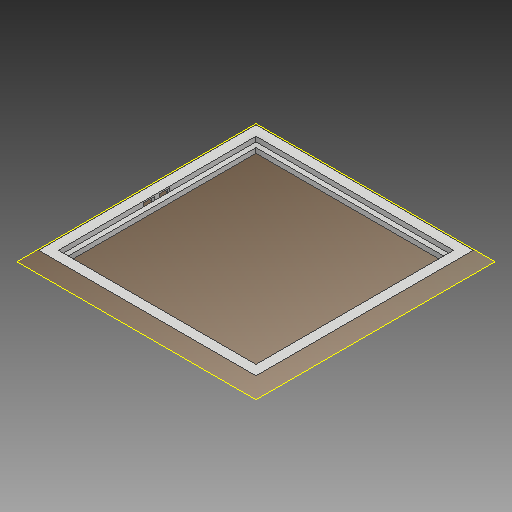
# Autodesk Inventor part: PV_Ramen_CPY
Saved by Autodesk Inventor 2018.2 (Build 222227000, 227)
## iProperties
Created: 2019-09-06
Part Number: PV_Ramen_CPY
Material: Generisch
Document SubType Name: Modeling
Designer: Lolob
Density: 1 g/cm^3
Appearance: Vorgabe
Author: DerLobre
Autodesk Inventor part; units mm, degrees
ref_plane "YZ Plane" through (0, 0, 0) normal (1, 0, 0) x (0, 1, 0)
ref_plane "XZ Plane" through (0, 0, 0) normal (0, 1, 0) x (-1, 0, 0)
ref_plane "XY Plane" through (0, 0, 0) normal (0, 0, 1) x (1, 0, 0)
sketch "Skizze1" plane through (0, 0, 0) normal (0, 0, 1) x (1, 0, 0)
  line L0 (-220, -220) -> (220, -220) projected
  line L1 (220, 220) -> (220, -220) projected
  line L2 (-220, 220) -> (-220, -220) projected
  line L3 (-220, 220) -> (220, 220) projected
  line L4 (200, 200) -> (-200, 200) projected
  line L5 (-200, 200) -> (-200, -200) projected
  line L6 (-200, -200) -> (200, -200) projected
  line L7 (200, -200) -> (200, 200) projected
  line L8 (220, -220) -> (-220, -220)
  line L9 (-220, -220) -> (-220, 220)
  line L10 (-220, 220) -> (220, 220)
  line L11 (220, 220) -> (220, -220)
  line L12 (200, -200) -> (-200, -200)
  line L13 (-200, -200) -> (-200, 200)
  line L14 (-200, 200) -> (200, 200)
  line L15 (200, 200) -> (200, -200)
  point P0 (0, 0)
  constraints: 16 end point, 4 parallel, 2 horizontal, 2 perpendicular
extrude "Extrusion1" add sketch "Skizze1" against normal blind 20
chamfer "Fase1" distance 20 angle 45 4 edges at (220, 0, -20) (0, 220, -20) (0, -220, -20) (-220, 0, -20)
ref_plane "Arbeitsebene1" through (0, 0, -20) normal (0, 0, 1) x (1, 0, 0)
sketch "Skizze3" plane through (0, 0, -20) normal (0, 0, 1) x (1, 0, 0)
  arc A0 (-205, 25.5) -> (-205, 4.5) centre (-205, 15) ccw projected
  arc A1 (-205, 25.5) -> (-205, 4.5) centre (-205, 15) ccw projected
  arc A2 (-205, -5.9522) -> (-205, -26.9522) centre (-205, -16.4522) ccw projected
  arc A3 (-205, -5.9522) -> (-205, -26.9522) centre (-205, -16.4522) ccw projected
  arc A4 (-205, -5.9522) -> (-205, -26.9522) centre (-205, -16.4522) ccw projected
  arc A5 (-205, -5.9522) -> (-205, -26.9522) centre (-205, -16.4522) ccw projected
  line L0 (-200, -26.9522) -> (-205, -26.9522) projected
  line L1 (-205, -5.9522) -> (-200, -5.9522) projected
  line L2 (-205, 4.5) -> (-200, 4.5)
  line L3 (-200, -200) -> (-200, 200) projected
  line L4 (-205, 25.5) -> (-200, 25.5)
  line L5 (-205, -5.9522) -> (-200, -5.9522)
  line L6 (-205, -26.9522) -> (-200, -26.9522)
  arc A6 (-205, 25.5) -> (-205, 4.5) centre (-205, 15) ccw
  arc A7 (-205, -5.9522) -> (-205, -26.9522) centre (-205, -16.4522) ccw
  point P0 (0, 0)
  constraints: 8 end point, 4 point on circle, 4 tangent, 2 centre point, 2 horizontal, 2 point on line, 1 parallel, 1 perpendicular
extrude "Extrusion2" cut sketch "Skizze3" along normal blind 17
sketch "Skizze5" plane through (0, 0, -20) normal (0, 0, 1) x (1, 0, 0)
  line L0 (-200, -26.9522) -> (-200, -200) projected
  line L1 (-200, -200) -> (200, -200) projected
  line L2 (200, -200) -> (200, 200) projected
  line L3 (-200, 200) -> (200, 200) projected
  line L4 (-200, -200) -> (200, -200)
  line L5 (200, -200) -> (200, 200)
  line L6 (200, 200) -> (-200, 200)
  line L7 (-200, 200) -> (-200, -200)
  line L8 (-190, -190) -> (190, -190)
  line L9 (190, -190) -> (190, 190)
  line L10 (190, 190) -> (-190, 190)
  line L11 (-190, 190) -> (-190, -190)
  point P0 (0, 0)
  dimension "d8" = 10
  dimension "d9" = 10
  dimension "d10" = 10
  dimension "d11" = 10
  constraints: 16 end point, 4 parallel, 2 horizontal, 2 perpendicular
  measures "d8" distance between parallel lines of L0 L11
  measures "d9" distance between parallel lines of L1 L8
  measures "d10" distance between parallel lines of L2 L9
  measures "d11" distance between parallel lines of L10 L3
extrude "Extrusion3" add sketch "Skizze5" along normal blind 10
